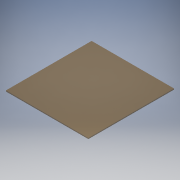
# Autodesk Inventor part: Roof
Saved by Autodesk Inventor 2016 (Build 200138000, 138)
## iProperties
Created: 2015-07-05
Part Number: Roof
Material: Polycarbonate, Smoke
Document SubType Name: Modeling
Designer: steele
Density: 1.2 g/cm^3
Appearance: Polycarbonate - Smoked
Author: steele
Autodesk Inventor part; units mm, degrees
ref_plane "YZ Plane" through (0, 0, 0) normal (1, 0, 0) x (0, 1, 0)
ref_plane "XZ Plane" through (0, 0, 0) normal (0, 1, 0) x (-1, 0, 0)
ref_plane "XY Plane" through (0, 0, 0) normal (0, 0, 1) x (1, 0, 0)
sketch "Sketch1" plane through (0, 0, 0) normal (0, 1, 0) x (-1, 0, 0)
  line L0 (-1079.5, 1122.3625) -> (-1079.5, -1122.3625)
  line L1 (-1079.5, -1122.3625) -> (1079.5, -1122.3625)
  line L2 (1079.5, -1122.3625) -> (1079.5, 1122.3625)
  line L3 (1079.5, 1122.3625) -> (-1079.5, 1122.3625)
  line L4 (-1079.5, 1122.3625) -> (1079.5, -1122.3625) construction
  line L5 (-1079.5, -1122.3625) -> (1079.5, 1122.3625) construction
  line L6 (-1079.5, 1122.3625) -> (1165.225, 1122.3625) construction
  point P0 (0, 0)
  dimension "d0" = 2244.725
  dimension "d1" = 90
  dimension "d2" = 2159
  constraints: 14 end point, 2 midpoint, 2 parallel, 2 perpendicular, 1 horizontal, 1 vertical
  measures "d0" distance of L0.start L0.end
  measures "d1" angle of L0 L6
  measures "d2" distance of L1.end L0.end
extrude "Extrusion1" add sketch "Sketch1" along normal blind 25.4
body "Solid1"
